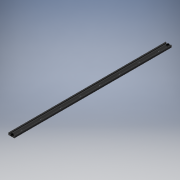
# Autodesk Inventor part: RSRR25-640
Saved by Autodesk Inventor 2019 (Build 230136000, 136)
## iProperties
Created: 2023-06-19
Part Number: RSRR25-640
Material: Generic
Catalog Web Link: www.cadenas.de
Description: RSRR-Roller Slide Rail
Vendor: MISUMI
Document SubType Name: Modeling
Designer: psAdmin
Manufacturer: MISUMI
Mass: 58.4433 g
Surface Area: 511.474 cm^2
Volume: 58.4433 cm^3
Density: 1 g/cm^3
Appearance: PSOLRGB-175-175-175
Category: PARTsolutions
Company: MISUMI
Title: RSRR25-640
Author: Cadenas PARTsolutions
Comments: Roller Slide Rail
PSOL_IDENT_0: {$CADENAS_DATA/23d-libs/misumi/metric/07_slide_rails/rsrr.prj},162 {VTYP=3D},{NB=RSRR25-640},{LINA=R
PSOL_IDENT_1: SRR25-640},{NN=RSRR},{DATE=29.05.2023 01:44:03},{GEOMDATE=16.07.2020 01:55:12},{VERSION=},{LINEID=10
PSOL_IDENT_2: },{WBVAR=LS},{WBNUMERIC=LS}  {NB=RSRR25-640},{LINA=RSRR25-640},{KT=DUMMY},{PN=RSRR25-640},{MAT=Alumi
PSOL_IDENT_3: num Alloy},{ST=Clear Anodizing},{NO=25},{LS=640},{NH=8},{LL=40},{RM=128},{LS1=160,240,320,400,480,56
PSOL_IDENT_4: 0,640,720,800,880,960,1040,1200},{T=RSRR}
NB: RSRR25-640
NN: RSRR
NT: Roller Slide Rail
NBSYN: $PN.
LINA: RSRR25-640
CATALOG: Misumi
PN: RSRR25-640
MAT: Aluminum Alloy
ST: Clear Anodizing
NO: 25
LS: 640
NH: 8
LL: 40
SUPPLIER: MISUMI
ARTICLENO: RSRR25-640
BOMINFO: RSRR25-640
CREATOR: CADENAS GmbH
Autodesk Inventor part; units mm, degrees
sketch "Sketch_1" plane through (0, 0, 0) normal (0, 0, 1) x (1, 0, 0)
  arc A0 (-12.5, 1) -> (-11.5, 0) centre (-11.5, 1) ccw
  line L0 (-11.5, 0) -> (11.5, 0)
  arc A1 (11.5, 0) -> (12.5, 1) centre (11.5, 1) ccw
  line L1 (12.5, 1) -> (12.5, 7.5)
  arc A2 (12.5, 7.5) -> (11.5, 8.5) centre (11.5, 7.5) ccw
  line L2 (11.5, 8.5) -> (9.5, 8.5)
  arc A3 (9.5, 8.5) -> (8.6036, 7.9432) centre (9.5, 7.5) ccw
  arc A4 (8.5, 3.4087) -> (8.6036, 7.9432) centre (7.5, 5.7) ccw
  line L3 (8.5, 3.4087) -> (8.5, 2.5)
  arc A5 (8, 2) -> (8.5, 2.5) centre (8, 2.5) ccw
  line L4 (8, 2) -> (-8, 2)
  arc A6 (-8.5, 2.5) -> (-8, 2) centre (-8, 2.5) ccw
  line L5 (-8.5, 2.5) -> (-8.5, 3.4087)
  arc A7 (-8.6036, 7.9432) -> (-8.5, 3.4087) centre (-7.5, 5.7) ccw
  arc A8 (-8.6036, 7.9432) -> (-9.5, 8.5) centre (-9.5, 7.5) ccw
  line L6 (-9.5, 8.5) -> (-11.5, 8.5)
  arc A9 (-11.5, 8.5) -> (-12.5, 7.5) centre (-11.5, 7.5) ccw
  line L7 (-12.5, 7.5) -> (-12.5, 1)
  constraints: 20 point on circle, 16 end point, 10 centre point
extrude "Extrusion1" add sketch "Sketch_1" along normal blind 640
sketch "Sketch_2" plane through (0, 0, 40) normal (0, 0, 1) x (1, 0, 0)
  line L0 (0, 0) -> (0, 2)
  line L1 (0, 2) -> (4.25, 2)
  line L2 (4.25, 2) -> (2.25, 0)
  line L3 (2.25, 0) -> (0, 0)
  line L4 (0, 0) -> (0, 2)
  constraints: 10 end point
revolve "Revolution1" cut sketch "Sketch_2" angle 360 about axis through (0, 0, 40) along (0, -1, 0)
pattern_linear "Rectangular Pattern1" count 8 spacing 80 along (0, 0, 1) of "Revolution1"
sketch "Sketch_4" plane through (0, 2, 0) normal (0, 1, 0) x (1, 0, 0)
  circle A0 centre (0, -3) radius 5
  constraints: 1 centre point
extrude "Extrusion2" add sketch "Sketch_4" along normal blind 5
sketch "Sketch_5" plane through (0, 2, 0) normal (0, 1, 0) x (1, 0, 0)
  circle A0 centre (0, -637) radius 5
  constraints: 1 centre point
extrude "Extrusion3" add sketch "Sketch_5" along normal blind 5
ref_plane "rail25_to_dummy_XY" through (0, 0, 320) normal (0, 0, 1) x (1, 0, 0)
ref_plane "rail25_to_dummy_YZ" through (0, 0, 320) normal (1, 0, 0) x (0, 1, 0)
ref_plane "rail25_to_dummy_ZX" through (0, 0, 320) normal (0, 1, 0) x (0, 0, 1)
ref_plane "to_slider_XY" through (0, 12, 320) normal (0, 0, 1) x (1, 0, 0)
ref_plane "to_slider_YZ" through (0, 12, 320) normal (1, 0, 0) x (0, 1, 0)
ref_plane "to_slider_ZX" through (0, 12, 320) normal (0, 1, 0) x (0, 0, 1)
body "Solid1"
